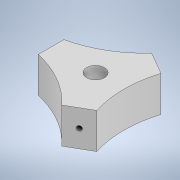
# Autodesk Inventor part: stability
Saved by Autodesk Inventor 2020 (Build 240168000, 168)
## iProperties
Created: 2019-07-11
Part Number: stability
Material: Generic
Document SubType Name: Modeling
Designer: ColinP
Density: 1 g/cm^3
Appearance: Default
Mass: 5.85901 g
Surface Area: 26.8401 cm^2
Volume: 5.85901 cm^3
Author: ColinP
Autodesk Inventor part; units mm, degrees
ref_plane "YZ Plane" through (0, 0, 0) normal (1, 0, 0) x (0, 1, 0)
ref_plane "XZ Plane" through (0, 0, 0) normal (0, 1, 0) x (-1, 0, 0)
ref_plane "XY Plane" through (0, 0, 0) normal (0, 0, 1) x (1, 0, 0)
sketch "Sketch1" plane through (0, 0, 0) normal (0, 1, 0) x (-1, 0, 0)
  line L0 (0, 0) -> (28.575, 0)
  line L1 (28.575, 0) -> (0, 0)
  line L2 (0, 0) -> (-14.2875, -24.7467)
  line L3 (0, 0) -> (28.575, 0) construction
  line L4 (0, 0) -> (-14.2875, 24.7467)
  line L5 (0, 0) -> (28.575, 0) construction
  circle A0 centre (28.575, 0) radius 2.54
  circle A1 centre (-14.2875, -24.7467) radius 2.54
  circle A2 centre (-14.2875, 24.7467) radius 2.54
  circle A3 centre (0, 0) radius 3.175
  circle A4 centre (0, 0) radius 6.35
  line L6 (-1.5875, -2.7496) -> (0, 0)
  line L7 (0, 0) -> (-6.35, 0)
  circle A5 centre (-14.2875, 24.7467) radius 3.81
  circle A6 centre (28.575, 0) radius 3.81
  circle A7 centre (-14.2875, -24.7467) radius 3.81
  line L8 (30.6811, 3.175) -> (-12.1814, 27.9217)
  line L9 (28.2054, -3.792) -> (-10.8187, -26.3226)
  line L10 (-18.0975, 24.7467) -> (-18.0975, -24.7467)
  line L11 (0, 0) -> (5.0525, -8.8146)
  line L12 (0, 0) -> (5.1463, 8.7602)
  line L13 (0, 0) -> (-10.16, 0)
  arc A8 (28.2054, -3.792) -> (-10.8187, -26.3226) centre (24.4473, -42.344) ccw
  arc A9 (-10.8187, 26.3226) -> (28.2054, 3.792) centre (24.4473, 42.344) ccw
  arc A10 (-17.3867, -22.5305) -> (-17.3867, 22.5305) centre (-48.8947, 0) ccw
  point P0 (5.1074, 8.7829)
  point P1 (-10.16, 0.0317)
  point P2 (30.2716, 3.4114)
  point P3 (28.2054, 3.792)
  point P4 (-10.8187, 26.3226)
  point P5 (-17.3867, 22.5305)
  point P6 (-17.3867, -22.5305)
  dimension "d9" = 6.35
  dimension "d41" = 12.7
  dimension "d0" = 28.575
  dimension "d1" = 28.575
  dimension "d2" = 120
  dimension "d3" = 28.575
  dimension "d4" = 120
  dimension "d5" = 5.08
  dimension "d6" = 5.08
  dimension "d7" = 5.08
  dimension "d42" = 7.62
  dimension "d43" = 7.62
  dimension "d44" = 7.62
  dimension "d47" = 10.16
  dimension "d48" = 10.16
  dimension "d49" = 10.16
  dimension "d52" = 360
  constraints: 28 end point, 15 point on circle, 9 centre point, 8 coincident, 4 horizontal, 3 tangent, 2 collinear, 2 equal length, 2 point on line, 1 horizontal alignment, 21 other
  measures "d0" distance of L0.start L0.end
  measures "d1" distance of L0.start L2.end
  measures "d2" angle of L2 L3
  measures "d3" distance of L0.start L4.end
  measures "d4" angle of L5 L4
  measures "d5" diameter of A0
  measures "d6" diameter of A1
  measures "d7" diameter of A2
  measures "d42" diameter of A5
  measures "d43" diameter of A6
  measures "d44" diameter of A7
  measures "d47" distance of L6.end L11.end
  measures "d48" distance of L6.end L12.end
  measures "d49" distance of L6.end L13.end
extrude "Extrusion4" add sketch "Sketch1" along normal blind 12.7 contours A3 L12 A4 L0 | L0 A4 L11 A3 | A3 L11 A4 L2 | L2 A4 L7 A3 | A3 L7 A4 L4 | L4 A4 L12 A3 | A4 L12 A9 A6 L0 | L0 A6 A8 L11 A4 | A4 L11 A8 A7 L2 | L2 A7 A10 L13 A4 | A4 L13 A10 A5 L4 | L4 A5 A9 L12 A4 | A6 L8 | A7 | A5 picked at (31.8987, 0.5122)
sketch "Sketch11" plane through (0, 12.7, 0) normal (0, 1, 0) x (1, 0, 0)
  arc A0 (10.8187, -26.3226) -> (-28.2054, -3.792) centre (-24.4473, -42.344) ccw projected
  arc A1 (17.3867, 22.5305) -> (17.3867, -22.5305) centre (48.8947, 0) ccw projected
  arc A2 (10.8187, -26.3226) -> (17.3867, -22.5305) centre (14.2875, -24.7467) ccw projected
  line L0 (0, 0) -> (14.2875, -24.7467)
  circle A3 centre (14.2875, -24.7467) radius 2.54 projected
  line L1 (14.2875, -24.7467) -> (8.2579, -14.3032)
  line L2 (14.2875, -24.7467) -> (7.9375, -13.7482)
  line L3 (7.9375, -13.7482) -> (11.895, -11.4633)
  line L4 (7.9375, -13.7482) -> (3.98, -16.033)
  circle A4 centre (14.2875, 24.7467) radius 2.54 projected
  line L5 (0, 0) -> (14.2875, 24.7467)
  line L6 (14.2875, 24.7467) -> (7.9375, 13.7482)
  line L7 (7.9375, 13.7482) -> (0, 0)
  circle A5 centre (-28.575, 0) radius 2.54 projected
  line L8 (0, 0) -> (-28.575, 0)
  line L9 (-28.575, 0) -> (-15.875, 0)
  line L10 (-15.875, 0) -> (-15.875, 4.5698)
  arc A6 (-28.2054, 3.792) -> (10.8187, 26.3226) centre (-24.4473, 42.344) ccw projected
  line L11 (-15.875, 0) -> (-15.875, -4.5698)
  line L12 (7.9375, 13.7482) -> (3.98, 16.033)
  line L13 (7.9375, 13.7482) -> (11.895, 11.4633)
  arc A7 (17.3867, 22.5305) -> (17.3867, -22.5305) centre (48.8947, 0) ccw projected
  arc A8 (-28.2054, 3.792) -> (-30.6811, -3.175) centre (-28.575, 0) ccw projected
  arc A9 (10.8187, -26.3226) -> (-28.2054, -3.792) centre (-24.4473, -42.344) ccw projected
  arc A10 (-30.2716, -3.4114) -> (-28.2054, -3.792) centre (-28.575, 0) ccw projected
  line L14 (-30.6811, -3.175) -> (-30.2716, -3.4114) projected
  arc A11 (17.3867, 22.5305) -> (10.8187, 26.3226) centre (14.2875, 24.7467) ccw projected
  point P0 (2.3124, -14.3387)
  point P1 (11.3663, -9.5918)
  point P2 (10.2682, -2.8934)
  point P3 (-3.012, -10.0809)
  dimension "d65" = 12.7
  dimension "d66" = 12.7
  dimension "d67" = 12.7
  constraints: 28 end point, 7 point on line, 5 point on circle, 3 perpendicular, 1 horizontal
  measures "d65" distance of L1.start L2.end
  measures "d66" distance of L5.end L6.end
  measures "d67" distance of L8.end L9.end
extrude "Extrusion6" cut sketch "Sketch11" against normal blind 25.4 contours A0 L4 L3 A1 A2 | A0 A10 L14 A8 A6 L10 L11 | L13 L12 A6 A11 A1
sketch "Sketch12" plane through (-15.875, 12.7, -4.5698) normal (-1, 0, 0) x (0, 0, 1)
  line L0 (0, -12.7) -> (0, 0) projected
  line L1 (0, -6.35) -> (9.0387, -6.35)
  line L2 (1.3948, 0) -> (7.7448, 0) projected
  line L3 (4.5698, 0) -> (4.5698, -12.7)
  line L4 (9.1395, -12.7) -> (20.6028, -12.7) projected
  line L5 (9.1395, 0) -> (20.6028, 0) projected
  line L6 (9.1395, -12.7) -> (9.1395, 0)
  line L7 (9.0387, -6.35) -> (9.1395, -6.35)
  line L8 (9.1395, 0) -> (9.1395, -12.7) projected
  point P0 (4.5698, -6.35)
  constraints: 8 end point, 4 midpoint, 2 vertical
sketch "Sketch13" plane through (11.895, 0, 11.4633) normal (0.5, 0, 0.8660254) x (0.8660254, 0, -0.5)
  line L0 (0, 12.7) -> (0, 0) projected
  line L1 (0, 6.35) -> (-9.1395, 6.35)
  line L2 (-9.1395, 0) -> (-9.1395, 12.7) projected
  line L3 (-9.1395, 12.7) -> (0, 12.7) projected
  line L4 (-4.5698, 12.7) -> (-4.5698, 0)
  point P0 (-4.5698, 6.35)
  constraints: 4 end point, 4 midpoint, 1 vertical
sketch "Sketch14" plane through (3.98, 0, -16.033) normal (0.5, 0, -0.8660254) x (-0.8660254, 0, -0.5)
  line L0 (-9.1395, 0) -> (-9.1395, 12.7) projected
  line L1 (-9.1395, 6.35) -> (0, 6.35)
  line L2 (0, 12.7) -> (0, 0) projected
  line L3 (-9.1395, 12.7) -> (0, 12.7) projected
  line L4 (-4.5698, 12.7) -> (-4.5698, 0)
  point P0 (-4.5698, 6.35)
  constraints: 4 end point, 4 midpoint, 1 vertical
hole "Hole5" at (7.9375, 6.35, 13.7482) direction (-0.5, 0, -0.8660254) diameter 1.6942 depth 6.6294 thread size "2-56 UNC" class "2B" standard "ANSI Unified Screw Threads"
hole "Hole6" at (-15.875, 6.35, 0) direction (1, 0, 0) diameter 1.6942 depth 6.6294 thread size "2-56 UNC" class "2B" standard "ANSI Unified Screw Threads"
hole "Hole7" at (7.9375, 6.35, -13.7482) direction (-0.5, 0, 0.8660254) diameter 1.6942 depth 6.6294 thread size "2-56 UNC" class "2B" standard "ANSI Unified Screw Threads"
body "Solid3"
